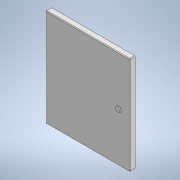
# Autodesk Inventor part: Door
Saved by Autodesk Inventor 2022 (Build 260153000, 153)
## iProperties
Created: 2024-10-27
Part Number: Door
Material: Ogólny
Document SubType Name: Modeling
Designer: NANOmatic
Density: 1 g/cm^3
Appearance: Domyślna
Author: NANOmatic
Autodesk Inventor part; units mm, degrees
ref_plane "YZ Plane" through (0, 0, 0) normal (1, 0, 0) x (0, 1, 0)
ref_plane "XZ Plane" through (0, 0, 0) normal (0, 1, 0) x (-1, 0, 0)
ref_plane "XY Plane" through (0, 0, 0) normal (0, 0, 1) x (1, 0, 0)
sketch "Szkic1" plane through (0, 0, 0) normal (0, 0, 1) x (1, 0, 0)
  line L0 (-150, 175) -> (150, 175)
  line L1 (150, 175) -> (150, -175)
  line L2 (150, -175) -> (-150, -175)
  line L3 (-150, -175) -> (-150, 175)
  line L4 (-150, 175) -> (150, -175) construction
  line L5 (150, 175) -> (-150, -175) construction
  point P0 (0, 0)
  dimension "d0" = 300
  dimension "d1" = 350
  constraints: 12 end point, 2 midpoint, 2 parallel, 1 horizontal, 1 perpendicular
  measures "d0" distance of L1.end L2.end
  measures "d1" distance of L0.end L1.end
extrude "Wyciągnięcie proste1" add sketch "Szkic1" against normal blind 19.15
sketch "Szkic4" plane through (0, 0, 0) normal (0, 0, 1) x (1, 0, 0)
  circle A0 centre (110, 0) radius 10
  line L0 (0, 0) -> (110, 0) construction
  dimension "d12" = 20
  dimension "d13" = 110
  constraints: 2 end point, 1 centre point, 1 horizontal
  measures "d12" diameter of A0
  measures "d13" distance of L0.start L0.end
extrude "Wyciągnięcie proste2" add sketch "Szkic4" along normal blind 3
chamfer "Faza1" distance 2 angle 45 1 edges at (100, 0, 3)
shell "Skorupa1" thickness 1.5 removed faces 1 at (-50, 58.3333, -19.15)
fillet "Zaokrąglenie1" radius 2.5 8 edges at (150, 175, -9.575) (-150, 175, -9.575) (-150, -175, -9.575) (150, -175, -9.575) (0, -175, 0) (150, 0, 0) (0, 175, 0) (-150, 0, 0)
sketch "Szkic2" plane through (0, 0, 0) normal (1, 0, 0) x (0, 1, 0)
  line L0 (173.5, -1.5) -> (-173.5, -1.5) projected
  arc A0 (151.5, -1.5) -> (163.5, -1.5) centre (157.5, -1.5) ccw
  line L1 (173.5, -1.5) -> (173.5, -19.15) projected
  point P0 (0, 0)
  dimension "d6" = 6
  dimension "d7" = 16
  constraints: 3 point on line, 2 point on circle, 1 centre point
  measures "d6" radius of A0
  measures "d7" distance from line of A0.centre L1
sketch "Szkic3" plane through (148.5, -173.5, -1.5) normal (0, 0, -1) x (-1, 0, 0)
  line L0 (271, 16) -> (26, 16)
  line L1 (16, 26) -> (16, 321)
  line L2 (26, 331) -> (271, 331)
  line L3 (281, 321) -> (281, 26)
  line L4 (281, 16) -> (16, 331) construction
  line L5 (16, 16) -> (281, 331) construction
  line L6 (0, 347) -> (297, 347) construction
  line L7 (297, 347) -> (281, 331) construction
  arc A0 (281, 321) -> (271, 331) centre (271, 321) ccw
  arc A1 (271, 16) -> (281, 26) centre (271, 26) ccw
  arc A2 (16, 26) -> (26, 16) centre (26, 26) ccw
  arc A3 (26, 331) -> (16, 321) centre (26, 321) ccw
  point P0 (148.5, 173.5)
  point P1 (148.5, 331)
  dimension "d8" = 22.6274
  dimension "d11" = 10
  constraints: 14 end point, 8 point on circle, 8 point on line, 8 tangent, 4 centre point, 3 equal radius, 3 midpoint, 2 parallel, 1 horizontal, 1 perpendicular
  measures "d8" distance of L6.end L5.end
  measures "d11" radius of A0
sweep "Przeciągnięcie1" add profiles "Szkic2" path "Szkic3"
sketch "Szkic5" plane through (0, 0, 0) normal (0, 1, 0) x (-1, 0, 0)
  line L0 (148.5, -19.15) -> (130.85, -1.5) construction
  line L1 (130.85, -1.5) -> (148.5, -1.5) construction
  line L2 (148.5, -1.5) -> (148.5, -19.15) construction
  point P0 (0, 0)
  point P1 (139.675, -10.325)
  constraints: 6 end point, 2 perpendicular, 1 horizontal, 1 midpoint
equation "\"d8\" = 1.41421 * d7"
